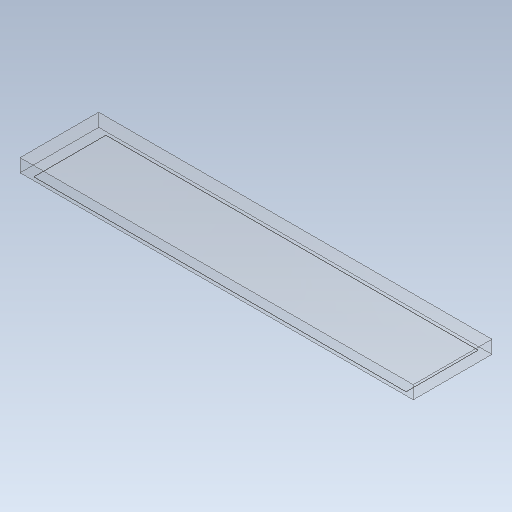
# Autodesk Inventor part: Acrylic Plate
Saved by Autodesk Inventor 2020.1 (Build 241239000, 239)
## iProperties
Created: 2019-07-22
Part Number: Acrylic Plate
Material: Polycarbonate, Clear
Document SubType Name: Modeling
Designer: Petar
Density: 1.2 g/cm^3
Appearance: Polycarbonate - Clear
Mass: 1.713 g
Surface Area: 17.3071 cm^2
Volume: 1.4275 cm^3
Author: Petar
Autodesk Inventor part; units mm, degrees
ref_plane "YZ Plane" through (0, 0, 0) normal (1, 0, 0) x (0, 1, 0)
ref_plane "XZ Plane" through (0, 0, 0) normal (0, 1, 0) x (-1, 0, 0)
ref_plane "XY Plane" through (0, 0, 0) normal (0, 0, 1) x (1, 0, 0)
sketch "Sketch1" plane through (0, 0, 0) normal (0, 1, 0) x (-1, 0, 0)
  line L0 (30, 6) -> (-30, 6)
  line L1 (-30, 6) -> (-30, -6)
  line L2 (-30, -6) -> (30, -6)
  line L3 (30, -6) -> (30, 6)
  line L4 (30, 6) -> (-30, -6) construction
  line L5 (-30, 6) -> (30, -6) construction
  point P0 (0, 0)
  dimension "d0" = 60
  dimension "d1" = 12
  constraints: 12 end point, 2 midpoint, 2 parallel, 1 horizontal, 1 perpendicular
  measures "d0" distance of L2.end L1.end
  measures "d1" distance of L1.end L0.end
extrude "Extrusion1" add sketch "Sketch1" along normal blind 2
sketch "Sketch2" plane through (0, 0, 0) normal (0, -1, 0) x (1, 0, 0)
  line L0 (28.4, 5.5) -> (-28.4, 5.5)
  line L1 (-28.4, 5.5) -> (-28.4, -5.5)
  line L2 (-28.4, -5.5) -> (28.4, -5.5)
  line L3 (28.4, -5.5) -> (28.4, 5.5)
  line L4 (28.4, 5.5) -> (-28.4, -5.5) construction
  line L5 (-28.4, 5.5) -> (28.4, -5.5) construction
  line L6 (30, -6) -> (-30, -6) construction
  line L7 (30, 6) -> (30, -6) construction
  point P0 (0, 0)
  dimension "d4" = 0.5
  dimension "d5" = 1.6
  constraints: 12 end point, 2 midpoint, 2 parallel, 1 horizontal, 1 perpendicular
  measures "d4" distance between parallel lines of L6 L2
  measures "d5" distance between parallel lines of L7 L3
extrude "Extrusion2" cut sketch "Sketch2" against normal blind 0.02
body "Solid1"
